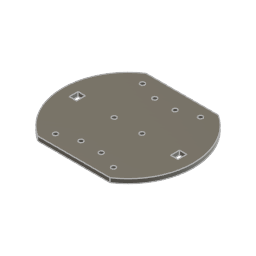
placa base (Autodesk Fusion 360 design; units mm, degrees)
part number: 2026-06-22-13-13-37-902
Autodesk Fusion 360 part; units mm, degrees
sketch "Boceto1" plane through (0, 0, 0) normal (0, 1, 0) x (1, 0, 0)
  line L0 (-24.9615, -37.4423) -> (24.9615, -37.4423)
  line L1 (24.9615, 37.4423) -> (-24.9615, 37.4423)
  arc A0 (24.9615, -37.4423) -> (24.9615, 37.4423) centre (0, 0) ccw
  arc A1 (-24.9615, 37.4423) -> (-24.9615, -37.4423) centre (0, 0) ccw
  circle A2 centre (-20.0139, -30.0084) radius 1.525
  circle A3 centre (-20.0295, 29.9916) radius 1.525
  circle A4 centre (19.9861, -29.9928) radius 1.525
  circle A5 centre (20.0133, 30.0074) radius 1.525
  circle A6 centre (-7, -25.4423) radius 1.525
  circle A7 centre (7, -25.4423) radius 1.525
  circle A8 centre (7, 25.4423) radius 1.525
  circle A9 centre (-7, 25.4423) radius 1.525
  circle A10 centre (-9.6, 0) radius 1.525
  circle A11 centre (9.6, 0) radius 1.525
  dimension "d2" = 40
  dimension "d3" = 60
  dimension "d4" = 3.05
  dimension "d5" = 3.05
  dimension "d6" = 3.05
  dimension "d7" = 3.05
  dimension "d15" = 14
  dimension "d16" = 3.05
  dimension "d17" = 3.05
  dimension "d19" = 14
  dimension "d20" = 3.05
  dimension "d21" = 3.05
  dimension "d34" = 3.05
  dimension "d36" = 3.05
  constraint coincident A0.centre A1.centre
  constraint horizontal L0
  constraint horizontal L1
  constraint concentric A0 A1
  measures "d2" distance of A2.centre A4.centre
  measures "d3" distance of A2.centre A3.centre
  measures "d4" diameter of A2
  measures "d5" diameter of A3
  measures "d6" diameter of A4
  measures "d7" diameter of A5
  measures "d15" distance of A6.centre A7.centre
  measures "d16" diameter of A6
  measures "d17" diameter of A7
  measures "d19" distance of A8.centre A9.centre
  measures "d20" diameter of A8
  measures "d21" diameter of A9
  measures "d34" diameter of A10
  measures "d36" diameter of A11
extrude "Extruir1" add sketch "Boceto1" along normal blind 4 contours L0 L1 A0 A1 | A10 | A11
sketch "Boceto2" plane through (0, 4, 0) normal (0, 1, 0) x (-1, 0, 0)
  circle A0 centre (7, -25.4423) radius 1.525
  arc A1 (24.9615, -37.4423) -> (24.9615, 37.4423) centre (0, 0) ccw
  line L0 (24.9615, 37.4423) -> (-24.9615, 37.4423)
  arc A2 (-24.9615, 37.4423) -> (-24.9615, -37.4423) centre (0, 0) ccw
  line L1 (-24.9615, -37.4423) -> (24.9615, -37.4423)
  circle A3 centre (-19.9861, 29.9928) radius 1.525
  circle A4 centre (20.0139, 30.0084) radius 1.525
  circle A5 centre (7, 25.4423) radius 1.525
  circle A6 centre (20.0295, -29.9916) radius 1.525
  circle A7 centre (-7, 25.4423) radius 1.525
  circle A8 centre (-7, -25.4423) radius 1.525
  circle A9 centre (-20.0133, -30.0074) radius 1.525
  line L2 (-32.5, 3) -> (-32.5, -3)
  line L3 (-32.5, -3) -> (-37.5, -3)
  line L4 (-37.5, -3) -> (-37.5, 3)
  line L5 (-37.5, 3) -> (-32.5, 3)
  line L6 (32.5, 3) -> (32.5, -3)
  line L7 (32.5, -3) -> (37.5, -3)
  line L8 (37.5, -3) -> (37.5, 3)
  line L9 (37.5, 3) -> (32.5, 3)
  dimension "d26" = 6
  dimension "d27" = 5
  dimension "d28" = 6
  dimension "d29" = 5
  constraint perpendicular L2 L3
  constraint perpendicular L3 L4
  constraint perpendicular L6 L7
  constraint perpendicular L7 L8
  measures "d26" distance of L2.start L2.end
  measures "d27" distance of L2.end L3.end
  measures "d28" distance of L6.start L6.end
  measures "d29" distance of L6.end L7.end
extrude "Extruir2" cut sketch "Boceto2" against normal blind 5 contours L2 L3 L4 L5 | L6 L7 L8 L9
extrude "Extruir3" cut sketch "Boceto1" along normal blind 12 contours A10 | A11
sketch "Boceto3" plane through (0, 4, 0) normal (0, 1, 0) x (-1, 0, 0)
  line L0 (32.5, -3) -> (32.5, 3)
  line L1 (32.5, 3) -> (37.5, 3)
  line L2 (37.5, 3) -> (37.5, -3)
  line L3 (37.5, -3) -> (32.5, -3)
  line L4 (-32.5, -3) -> (-37.5, -3)
  line L5 (-37.5, -3) -> (-37.5, 3)
  line L6 (-37.5, 3) -> (-32.5, 3)
  line L7 (-32.5, 3) -> (-32.5, -3)
  arc A0 (24.9615, -37.4423) -> (24.9615, 37.4423) centre (0, 0) ccw
  line L8 (24.9615, 37.4423) -> (-24.9615, 37.4423)
  arc A1 (-24.9615, 37.4423) -> (-24.9615, -37.4423) centre (0, 0) ccw
  line L9 (-24.9615, -37.4423) -> (24.9615, -37.4423)
  circle A2 centre (-20.0133, -30.0074) radius 1.525
  circle A3 centre (-19.9861, 29.9928) radius 1.525
  circle A4 centre (-7, -25.4423) radius 1.525
  circle A5 centre (7, -25.4423) radius 1.525
  circle A6 centre (7, 25.4423) radius 1.525
  circle A7 centre (-7, 25.4423) radius 1.525
  circle A8 centre (20.0139, 30.0084) radius 1.525
  circle A9 centre (20.0295, -29.9916) radius 1.525
  circle A10 centre (-9.6, 0) radius 1.525
  circle A11 centre (9.6, 0) radius 1.525
  circle A12 centre (7, -25.4423) radius 1.525
  circle A13 centre (20.0295, -29.9916) radius 1.525
  circle A14 centre (-7, -25.4423) radius 1.525
  circle A15 centre (-20.0133, -30.0074) radius 1.525
  circle A16 centre (20.0139, 30.0084) radius 1.525
  circle A17 centre (7, 25.4423) radius 1.525
  circle A18 centre (-7, 25.4423) radius 1.525
  circle A19 centre (-19.9861, 29.9928) radius 1.525
  line L10 (37.5, -3) -> (32.5, -3)
  line L11 (32.5, -3) -> (32.5, 3)
  line L12 (32.5, 3) -> (37.5, 3)
  line L13 (37.5, 3) -> (37.5, -3)
  line L14 (-32.5, -3) -> (-37.5, -3)
  line L15 (-37.5, -3) -> (-37.5, 3)
  line L16 (-37.5, 3) -> (-32.5, 3)
  line L17 (-32.5, 3) -> (-32.5, -3)
  line L18 (24.9615, 37.4423) -> (-24.9615, 37.4423)
  line L19 (24.9615, -37.4423) -> (-24.9615, -37.4423)
  arc A20 (24.9615, -37.4423) -> (24.9615, 37.4423) centre (0, 0) ccw
  arc A21 (-24.9615, 37.4423) -> (-24.9615, -37.4423) centre (0, 0) ccw
  circle A22 centre (0, -9.6) radius 1.525
  circle A23 centre (0, 9.6) radius 1.525
  dimension "d42" = 3.05
  dimension "d43" = 3.05
  dimension "d44" = 3.05
  dimension "d45" = 3.05
  dimension "d46" = 3.05
  dimension "d47" = 3.05
  dimension "d48" = 3.05
  dimension "d49" = 3.05
  dimension "d52" = 3.05
  dimension "d53" = 3.05
  constraint concentric A5 A12
  constraint concentric A9 A13
  constraint concentric A4 A14
  constraint concentric A2 A15
  constraint concentric A8 A16
  constraint concentric A6 A17
  constraint concentric A7 A18
  constraint concentric A3 A19
  constraint coincident L2.end L3.start
  constraint coincident L0.start L3.end
  constraint coincident L0.end L1.start
  constraint coincident L1.end L2.start
  constraint coincident L4.start L7.end
  constraint coincident L4.end L5.start
  constraint coincident L5.end L6.start
  constraint coincident L6.end L7.start
  constraint concentric A0 A20
  constraint coincident A0.end L8.start
  constraint coincident L8.end A1.start
  constraint coincident A0.start L9.end
  constraint coincident A1.end L9.start
  constraint concentric A20 A21
  constraint coincident A0.centre A1.centre
  measures "d42" diameter of A12
  measures "d43" diameter of A13
  measures "d44" diameter of A14
  measures "d45" diameter of A15
  measures "d46" diameter of A16
  measures "d47" diameter of A17
  measures "d48" diameter of A18
  measures "d49" diameter of A19
  measures "d52" diameter of A22
  measures "d53" diameter of A23
move_face "CarasDesfase1" offset -1 1 faces at (21.0321, 0, -10.8988)
